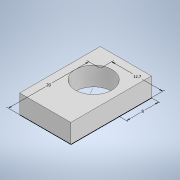
# Autodesk Inventor part: chapa
Saved by Autodesk Inventor 2021 (Build 250183000, 183)
## iProperties
Created: 2026-06-09
Part Number: chapa
Material: Generic
Document SubType Name: Sheet Metal
Designer: nelso
Density: 1 g/cm^3
Sheet Metal Rule: Default_mm
Appearance: Default
Author: nelso
Autodesk Inventor part; units mm, degrees
ref_plane "YZ Plane" through (0, 0, 0) normal (1, 0, 0) x (0, 1, 0)
ref_plane "XZ Plane" through (0, 0, 0) normal (0, 1, 0) x (-1, 0, 0)
ref_plane "XY Plane" through (0, 0, 0) normal (0, 0, 1) x (1, 0, 0)
sketch "Sketch1" plane through (0, 0, 0) normal (0, 1, 0) x (-1, 0, 0)
  line L0 (-6.35, 10) -> (6.35, 10)
  line L1 (6.35, 10) -> (6.35, -10)
  line L2 (6.35, -10) -> (-6.35, -10)
  line L3 (-6.35, -10) -> (-6.35, 10)
  line L4 (-6.35, 10) -> (6.35, -10) construction
  line L5 (6.35, 10) -> (-6.35, -10) construction
  line L6 (-6.35, -10) -> (-6.35, -2)
  line L7 (-6.35, -2) -> (0, -2)
  point P0 (0, 0)
  dimension "d0" = 12.7
  dimension "d1" = 20
  dimension "d2" = 8
  constraints: 16 end point, 2 midpoint, 2 parallel, 2 perpendicular, 1 coincident, 1 horizontal, 1 point on line
  measures "d0" distance of L1.end L2.end
  measures "d1" distance of L0.end L1.end
  measures "d2" distance of L2.end L6.end
extrude "Plate1" add sketch "Sketch1" along normal blind 4.7
hole "Hole1" at (0, 0, -2) direction (0, 1, 0) diameter 9 end through all clearance for "Countersunk Flat Head Screw ISO 2009/7046" size "M8" standard "ISO"
equation "\"d9\" = Thickness"
equation "\"d3\" = Thickness"
equation "\"BendRadius\" = Thickness"
equation "\"BendReliefWidth\" = Thickness"
equation "\"BendReliefDepth\" = 0.5 * Thickness"
equation "\"CornerReliefSize\" = 4 * Thickness"
equation "\"MinimumRemnant\" = 2 * Thickness"
equation "\"TransitionRadius\" = BendRadius"
equation "\"JacobiRadiusSize\" = BendRadius"
equation "\"GapSize\" = Thickness"
equation "\"Thickness\" = 4.7"
body "Solid1"
